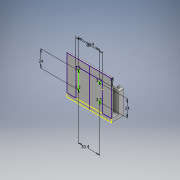
# Autodesk Inventor part: px4 Flow Mount
Saved by Autodesk Inventor 2018 (Build 220112000, 112)
## iProperties
Created: 2017-07-06
Part Number: px4 Flow Mount
Material: Generic
Document SubType Name: Modeling
Designer: klyu
Density: 1 g/cm^3
Appearance: Default
Author: klyu
Autodesk Inventor part; units mm, degrees
ref_plane "YZ Plane" through (0, 0, 0) normal (1, 0, 0) x (0, 1, 0)
ref_plane "XZ Plane" through (0, 0, 0) normal (0, 1, 0) x (-1, 0, 0)
ref_plane "XY Plane" through (0, 0, 0) normal (0, 0, 1) x (1, 0, 0)
sketch "Sketch1" plane through (0, 0, 0) normal (0, 1, 0) x (-1, 0, 0)
  line L0 (0, 0) -> (4.5, 0)
  line L1 (4.5, 0) -> (4.5, -20)
  line L2 (4.5, -20) -> (0, -20)
  line L3 (0, -20) -> (0, 0)
  line L4 (34, 0) -> (38.5, 0)
  line L5 (38.5, 0) -> (38.5, -20)
  line L6 (38.5, -20) -> (34, -20)
  line L7 (34, -20) -> (34, 0)
  line L8 (51.25, 0) -> (-12.75, 0)
  line L9 (-12.75, 0) -> (-12.75, -25)
  line L10 (-12.75, -25) -> (51.25, -25)
  line L11 (51.25, -25) -> (51.25, 0)
  line L12 (19.25, 0) -> (19.25, -42)
  dimension "d0" = 4.5
  dimension "d1" = 20
  dimension "d2" = 4.5
  dimension "d3" = 20
  dimension "d4" = 38.5
  dimension "d5" = 25
  dimension "d6" = 64
  dimension "d7" = 14.75
  dimension "d8" = 32
  constraints: 26 end point, 6 parallel, 3 horizontal, 3 perpendicular, 2 collinear, 1 midpoint, 1 vertical
  measures "d0" distance between parallel lines of L1 L3
  measures "d1" distance between parallel lines of L2 L0
  measures "d2" distance between parallel lines of L5 L7
  measures "d3" distance between parallel lines of L6 L4
  measures "d4" distance between parallel lines of L3 L5
  measures "d5" distance between parallel lines of L10 L8
  measures "d6" distance between parallel lines of L9 L11
  measures "d7" distance between parallel lines of L12 L7
  measures "d8" distance between parallel lines of L12 L11
extrude "Extrusion1" add sketch "Sketch1" along normal blind 2 contours L3 L2 L1 L8 L12 L10 L9 | L8 L7 L6 L5 L11 L10 L12
sketch "Sketch2" plane through (0, 2, 0) normal (0, 1, 0) x (1, 0, 0)
  line L0 (0, 0) -> (12.75, 0) projected
  line L1 (12.75, 0) -> (10.75, 0)
  line L2 (10.75, 0) -> (10.75, 25)
  line L3 (10.75, 25) -> (12.75, 25)
  line L4 (12.75, 25) -> (12.75, 0)
  line L5 (12.75, 25) -> (-51.25, 25) projected
  line L6 (-49.25, 0) -> (-51.25, 0)
  line L7 (-51.25, 0) -> (-51.25, 25)
  line L8 (-51.25, 25) -> (-49.25, 25)
  line L9 (-49.25, 25) -> (-49.25, 0)
  line L10 (-51.25, 25) -> (-51.25, 0) projected
  line L11 (-51.25, 0) -> (-38.5, 0) projected
  point P0 (13.75, 26)
  dimension "d11" = 2
  dimension "d12" = 2
  constraints: 14 end point, 4 collinear, 3 parallel, 2 horizontal, 2 perpendicular, 1 vertical, 3 other
  measures "d11" distance between parallel lines of L4 L2
extrude "Extrusion2" add sketch "Sketch2" along normal blind 3
sketch "Sketch3" plane through (0, 5, 0) normal (0, 1, 0) x (1, 0, 0)
  line L0 (-51.25, 0) -> (-44.25, 0)
  line L1 (-44.25, 0) -> (-44.25, 25)
  line L2 (-44.25, 25) -> (-51.25, 25)
  line L3 (-51.25, 25) -> (-51.25, 0)
  line L4 (12.75, 0) -> (12.75, 25) projected
  line L5 (12.75, 0) -> (5.75, 0)
  line L6 (5.75, 0) -> (5.75, 25)
  line L7 (5.75, 25) -> (12.75, 25)
  line L8 (12.75, 25) -> (12.75, 0)
  line L9 (10.75, 25) -> (-49.25, 25) projected
  point P0 (0, 0)
  dimension "d15" = 7
  dimension "d16" = 7
  constraints: 16 end point, 4 parallel, 2 horizontal, 2 perpendicular, 1 collinear, 1 point on line
  measures "d15" distance between parallel lines of L3 L1
  measures "d16" distance between parallel lines of L4 L6
extrude "Extrusion3" add sketch "Sketch3" along normal blind 2
sketch "Sketch8" plane through (0, 0, 0) normal (0, -1, 0) x (1, 0, 0)
  line L0 (12.75, -3) -> (-51.25, -3)
  line L1 (-51.25, -3) -> (-51.25, 0)
  line L2 (-51.25, 0) -> (12.75, 0)
  line L3 (12.75, 0) -> (12.75, -3)
  line L4 (12.75, 0) -> (12.75, -25) projected
  line L5 (-51.25, -25) -> (-51.25, 0) projected
  line L6 (-34, 0) -> (-4.5, 0) projected
  point P0 (0, 0)
  point P1 (12.75, -95)
  point P2 (-51.25, -95)
  dimension "d45" = 3
  constraints: 8 end point, 3 collinear, 3 perpendicular, 1 horizontal
  measures "d45" distance between parallel lines of L2 L0
extrude "Extrusion7" add sketch "Sketch8" against normal up to surface (2 mm away)
fillet "Fillet1" radius 2 8 edges at (12.75, 3.5, 0) (-51.25, 3.5, 0) (-44.25, 6, 0) (5.75, 6, 0) (0, 1, -20) (-38.5, 1, -20) (0, 1, -3) (-38.5, 1, -3)
sketch "Sketch9" plane through (0, 2, 0) normal (0, 1, 0) x (1, 0, 0)
  line L0 (-36.5, 3) -> (-34, 3) projected
  line L1 (-34, 3) -> (-33.5, 3)
  line L2 (-33.5, 3) -> (-33.5, 20)
  line L3 (-33.5, 20) -> (-34, 20)
  line L4 (-4.5, 3) -> (-2, 3) projected
  line L5 (-4.5, 3) -> (-5, 3)
  line L6 (-5, 3) -> (-5, 20)
  line L7 (-4.5, 20) -> (-2, 20) projected
  line L8 (-5, 20) -> (-4.5, 20)
  line L9 (-4.5, 3) -> (-4.5, 20) projected
  line L10 (-34, 20) -> (-34, 3) projected
  point P0 (0, 0)
  dimension "d48" = 0.5
  dimension "d49" = 0.5
  constraints: 12 end point, 4 perpendicular, 2 horizontal, 1 coincident
  measures "d48" distance between parallel lines of L9 L6
  measures "d49" distance between parallel lines of L10 L2
extrude "Extrusion8" cut sketch "Sketch9" against normal through all
sketch "Sketch10" plane through (12.75, 0, -25) normal (0, 0, -1) x (-1, 0, 0)
  line L0 (0, 7) -> (7, 7) projected
  line L1 (64, 0) -> (64, 7) projected
  line L2 (0, 7) -> (64, 7)
  line L3 (64, 7) -> (64, 0)
  line L4 (64, 0) -> (0, 0)
  line L5 (0, 0) -> (0, 7)
  point P0 (12.75, 0)
  constraints: 8 end point, 2 parallel, 1 horizontal, 1 perpendicular
extrude "Extrusion9" add sketch "Sketch10" along normal blind 10
sketch "Sketch11" plane through (0, 0, 0) normal (0, -1, 0) x (1, 0, 0)
  line L0 (-51.25, -2) -> (-51.25, -35) projected
  line L1 (12.75, -2) -> (12.75, -35) projected
  line L2 (-51.25, -35) -> (12.75, -35)
  line L3 (12.75, -35) -> (12.75, -30)
  line L4 (12.75, -30) -> (-51.25, -30)
  line L5 (-51.25, -30) -> (-51.25, -35)
  point P0 (0, 0)
  dimension "d54" = 5
  constraints: 8 end point, 2 parallel, 1 horizontal, 1 perpendicular, 1 point on line
  measures "d54" distance between parallel lines of L2 L4
extrude "Extrusion10" add sketch "Sketch11" along normal blind 10
sketch "Sketch12" plane through (-51.25, 0, -30) normal (0, 0, 1) x (1, 0, 0)
  line L0 (0, 7) -> (0, -10) projected
  line L1 (0, -10) -> (64, -10)
  line L2 (64, -10) -> (64, -8)
  line L3 (64, -8) -> (0, -8)
  line L4 (0, -8) -> (0, -10)
  point P0 (51.25, 0)
  dimension "d57" = 2
  constraints: 8 end point, 2 parallel, 1 horizontal, 1 perpendicular
  measures "d57" distance between parallel lines of L3 L1
extrude "Extrusion11" add sketch "Sketch12" along normal blind 50
sketch "Sketch13" plane through (0, -10, 0) normal (0, -1, 0) x (1, 0, 0)
  line L0 (-38.25, -30) -> (-38.25, 10)
  line L1 (-0.25, 10) -> (-0.25, -30)
  line L2 (-38.25, 10) -> (-0.25, 10)
  circle A0 centre (-34.7601, -18) radius 1.65
  circle A1 centre (-4.3601, 6) radius 1.65
  circle A2 centre (-4.3601, -18) radius 1.65
  circle A3 centre (-34.7601, 6) radius 1.65
  line L3 (-0.25, -30) -> (12.75, -30)
  line L4 (-34.7601, -18) -> (-34.7601, 6)
  line L5 (-38.25, -30) -> (-51.25, -30)
  line L6 (-51.25, -30) -> (-51.25, 20)
  line L7 (-51.25, 20) -> (12.75, 20)
  line L8 (12.75, 20) -> (12.75, -30)
  line L9 (12.75, -35) -> (12.75, 20) projected
  line L10 (-51.25, -35) -> (-51.25, 20) projected
  line L11 (-51.25, 20) -> (12.75, 20) projected
  line L12 (-51.25, -30) -> (12.75, -30) projected
  line L13 (-51.25, -35) -> (12.75, -35) projected
  line L14 (-51.25, -35) -> (12.75, -35) projected
  line L15 (-19.25, -35) -> (-19.25, 20)
  line L16 (12.75, 20) -> (-51.25, 20) projected
  point P0 (0, 0)
  dimension "d60" = 38
  dimension "d61" = 3.3
  dimension "d62" = 3.3
  dimension "d63" = 3.3
  dimension "d64" = 3.3
  dimension "d68" = 30.4
  dimension "d69" = 24
  dimension "d70" = 24
  dimension "d71" = 30.4
  dimension "d76" = 10
  constraints: 20 end point, 5 collinear, 4 centre point, 3 horizontal, 3 vertical, 2 midpoint, 2 perpendicular, 1 other
  measures "d60" distance between parallel lines of L1 L0
  measures "d61" diameter of A0
  measures "d62" diameter of A1
  measures "d63" diameter of A2
  measures "d64" diameter of A3
  measures "d68" distance of L4.end A1.centre
  measures "d69" distance of A1.centre A2.centre
  measures "d70" distance of L4.end L4.start
  measures "d71" distance of A2.centre L4.start
  measures "d76" distance between parallel lines of L7 L2
body "Solid1"
